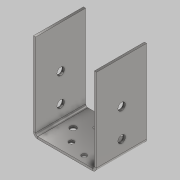
# Autodesk Inventor part: RR-PCSS-W3M2
Saved by Autodesk Inventor 2021 (Build 250183000, 183)
## iProperties
Created: 2021-09-22
Part Number: RR-PCSS-W3M2
Material: Stal nierdzewna
Document SubType Name: Konstrukcja blachowa
Designer: Marcin Sobczak
Density: 8 g/cm^3
Sheet Metal Rule: Domyślny_mm
Appearance: Częściowo polerowana
Flat Pattern Width: 4.43 cm
Flat Pattern Length: 20.3848 cm
Flat Pattern Area: 90.3046 cm^2
Sheet Metal Width: 44,300 mm
Sheet Metal Length: 203,848 mm
Sheet Metal Area: 9030,457 mm^2
Project: Ramie robotyczne
Mass: 140.956 g
Surface Area: 188.801 cm^2
Volume: 17.6196 cm^3
Author: marci
Title: Łącznik elementów 3M2
Autodesk Inventor part; units mm, degrees
note: some values were not read from the file. Chosen so that the rebuilt part matches the saved one: direction of "Otwór4"; direction of "Otwór5".
ref_plane "YZ Plane" through (0, 0, 0) normal (1, 0, 0) x (0, 1, 0)
ref_plane "XZ Plane" through (0, 0, 0) normal (0, 1, 0) x (-1, 0, 0)
ref_plane "XY Plane" through (0, 0, 0) normal (0, 0, 1) x (1, 0, 0)
sketch "Szkic1" plane through (0, 0, 0) normal (0, 1, 0) x (-1, 0, 0)
  line L0 (-28, -22.15) -> (28, -22.15)
  line L1 (28, -22.15) -> (28, 22.15)
  line L2 (28, 22.15) -> (-28, 22.15)
  line L3 (-28, 22.15) -> (-28, -22.15)
  line L4 (-28, -22.15) -> (28, 22.15) construction
  line L5 (28, -22.15) -> (-28, 22.15) construction
  point P0 (0, 0)
  dimension "d0" = 56
  dimension "d1" = 44.3
  measures "d0" distance of L2.end L1.end
  measures "d1" distance of L1.end L0.end
extrude "Płyta1" add sketch "Szkic1" along normal blind 2
sketch "Szkic4" plane through (26, 0, -22.15) normal (1, 0, 0) x (0, 1, 0)
  line L0 (0, 44.3) -> (0, 0)
  line L1 (0, 0) -> (77.4, 0)
  line L2 (77.4, 0) -> (77.4, 44.3)
  line L3 (77.4, 44.3) -> (0, 44.3)
  constraints: 6 end point, 1 horizontal, 1 perpendicular, 1 vertical
edge flange "Kołnierz3" height 77.4 angle 90 thickness 2 bend radius 2 thickness toward (1, 0, 0) relief tear relief width 2 relief depth 1 corner gap 2 corner form 0 edges at (28, 2, 0) (-28, 2, 0) wall of the first edge with corners at (26, 0, 22.15) (26, 0, -22.15) (26, 77.4, -22.15) (26, 77.4, 22.15)
bend "Zagięcie3"
corner "Narożnik3"
sketch "Szkic9" plane through (-28, 77.4, -22.15) normal (-1, 0, 0) x (0, 0, 1)
  point P0 (22.15, -37.4)
  point P1 (22.15, -62.4)
hole "Otwór4" at (-28, 40, 0) at (-28, 15, 0) direction (1, 0, 0) diameter 6.6 depth 2
sketch "Szkic10" plane through (26, 77.4, -22.15) normal (-1, 0, 0) x (0, 0, 1)
  point P0 (22.15, -37.4)
  point P1 (22.15, -62.4)
hole "Otwór5" at (26, 40, 0) at (26, 15, 0) direction (1, 0, 0) diameter 6.6 depth 2
sketch "Szkic11" plane through (0, 2, 0) normal (0, 1, 0) x (1, 0, 0)
  point P0 (11, -16.15)
  point P1 (11, 16.35)
hole "Otwór6" at (11, 2, 16.15) at (11, 2, -16.35) direction (0, -1, 0) diameter 4.5 end through all
sketch "Szkic12" plane through (0, 2, 0) normal (0, 1, 0) x (1, 0, 0)
  point P0 (-5, 10.5981)
  point P1 (-5, -11.4019)
hole "Otwór7" at (-5, 2, -10.5981) at (-5, 2, 11.4019) direction (0, -1, 0) diameter 4.5 end through all
sketch "Szkic13" plane through (0, 2, 0) normal (0, 1, 0) x (1, 0, 0)
  point P0 (-15, 0.1)
hole "Otwór8" at (-15, 2, -0.1) direction (0, -1, 0) diameter 5.5 end through all
equation "\"d2\" = Grubość"
equation "\"d23\" = SzerokośćGięciaPodcięcia"
equation "\"d24\" = GłębokośćGięciaPodcięcia"
equation "\"d25\" = MinimalnaPozostałość"
equation "\"d26\" = PromieńPrzejścia"
equation "\"d29\" = PromieńGięcia"
equation "\"d30\" = RozmiarPodcięciaNarożnika"
equation "\"d31\" = Wielk_odstępu"
equation "\"d32\" = Rozmiar_promienia_Jacobiego"
equation "\"PromieńGięcia\" = Grubość"
equation "\"SzerokośćGięciaPodcięcia\" = Grubość"
equation "\"GłębokośćGięciaPodcięcia\" = 0.5 * Grubość"
equation "\"RozmiarPodcięciaNarożnika\" = 4 * Grubość"
equation "\"MinimalnaPozostałość\" = 2 * Grubość"
equation "\"PromieńPrzejścia\" = PromieńGięcia"
equation "\"Rozmiar_promienia_Jacobiego\" = PromieńGięcia"
equation "\"Wielk_odstępu\" = Grubość"
equation "\"Grubość\" = 2"
